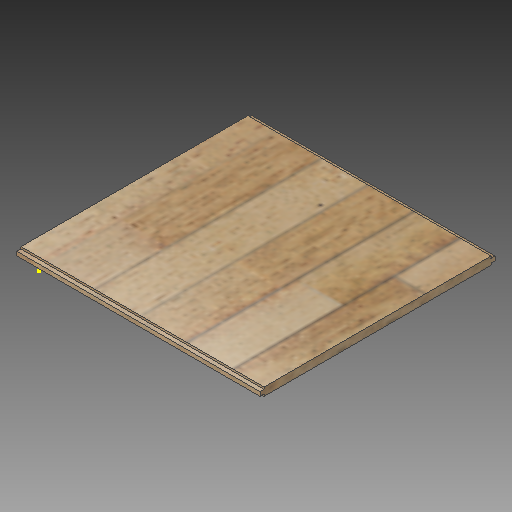
# Autodesk Inventor part: Bauteil3
Saved by Autodesk Inventor 2019 (Build 230136000, 136)
## iProperties
Created: 2021-09-26
Part Number: Bauteil3
Material: Holz (Ahorn)
Document SubType Name: Modeling
Designer: mritt
Density: 0.67 g/cm^3
Appearance: Ahorn - natur - glänzend - dunkel getönt
Author: mritt
Autodesk Inventor part; units mm, degrees
ref_plane "YZ Plane" through (0, 0, 0) normal (1, 0, 0) x (0, 1, 0)
ref_plane "XZ Plane" through (0, 0, 0) normal (0, 1, 0) x (-1, 0, 0)
ref_plane "XY Plane" through (0, 0, 0) normal (0, 0, 1) x (1, 0, 0)
sketch "Skizze2" plane through (0, 0, 0) normal (0, 1, 0) x (-1, 0, 0)
  line L0 (27.6477, 247.101) -> (-272.3523, 247.101)
  line L1 (-272.3523, 247.101) -> (-272.3523, -42.899)
  line L2 (-272.3523, -42.899) -> (27.6477, -42.899)
  line L3 (27.6477, -42.899) -> (27.6477, 247.101)
  point P0 (0, 0)
  dimension "d1" = 290
  dimension "d2" = 300
  constraints: 8 end point, 2 parallel, 1 horizontal, 1 perpendicular
  measures "d1" distance of L2.end L0.start
  measures "d2" distance of L1.end L2.end
extrude "Extrusion1" add sketch "Skizze2" along normal blind 10
sketch "Skizze3" plane through (-27.6477, 0, 247.101) normal (0, 0, 1) x (1, 0, 0)
  point P0 (27.6477, 0)
sketch "Skizze4" plane through (-27.6477, 0, 247.101) normal (0, 0, 1) x (1, 0, 0)
  line L0 (0, 10) -> (300, 10) projected
  line L1 (0, 0) -> (0, 10) projected
  line L2 (300, 0) -> (300, 10) projected
  line L3 (0, 7.5) -> (300, 7.5)
  line L4 (300, 7.5) -> (300, 2.5)
  line L5 (300, 2.5) -> (0, 2.5)
  line L6 (0, 2.5) -> (0, 7.5)
  line L7 (0, 0) -> (300, 0) projected
  line L8 (0, 10) -> (300, 10)
  line L9 (300, 10) -> (300, 0)
  line L10 (300, 0) -> (0, 0)
  line L11 (0, 0) -> (0, 10)
  dimension "d8" = 2.5
  dimension "d9" = 2.5
  constraints: 16 end point, 4 parallel, 2 horizontal, 2 perpendicular, 2 point on line
  measures "d8" distance between parallel lines of L0 L3
  measures "d9" distance between parallel lines of L5 L7
extrude "Extrusion2" cut sketch "Skizze4" against normal blind 5 contours L0 L2 L3 L1 | L5 L2 L7 L1
sketch "Skizze5" plane through (272.3523, 0, -42.899) normal (0, 0, -1) x (-1, 0, 0)
  line L0 (0, 0) -> (0, 10) projected
  line L1 (0, 7.5) -> (300, 7.5)
  line L2 (300, 7.5) -> (300, 2.5)
  line L3 (300, 2.5) -> (0, 2.5)
  line L4 (0, 2.5) -> (0, 7.5)
  line L5 (0, 10) -> (300, 10) projected
  line L6 (0, 0) -> (300, 0) projected
  line L7 (300, 10) -> (0, 10) projected
  line L8 (300, 10) -> (0, 10)
  line L9 (0, 10) -> (0, 0)
  line L10 (0, 0) -> (300, 0)
  line L11 (300, 0) -> (300, 10)
  point P0 (272.3523, 0)
  dimension "d12" = 2.5
  dimension "d13" = 2.5
  constraints: 16 end point, 4 parallel, 2 horizontal, 2 perpendicular, 1 point on line
  measures "d12" distance between parallel lines of L5 L1
  measures "d13" distance between parallel lines of L6 L3
extrude "Extrusion3" cut sketch "Skizze5" against normal blind 5 contours L0 L3 L11 L6 | L0 L5 L11 L1
